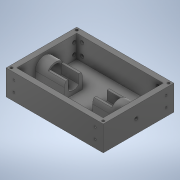
# Autodesk Inventor part: BodyWedgeBaseV3.1
Saved by Autodesk Inventor 2020 (Build 240168000, 168)
## iProperties
Created: 2023-11-26
Part Number: BodyWedgeBaseV3.1
Material: Thermoplastic Resin
Document SubType Name: Modeling
Designer: smz3rm
Density: 1.28 g/cm^3
Appearance: Smooth - Black
Mass: 119.612 g
Surface Area: 420.017 cm^2
Volume: 93.4466 cm^3
SideThickness: 6.000 mm
BaseThickness: 3.000 mm
TopThickness: 1.588 mm
BoxWidth: 110.000 mm
BoxLength: 80.000 mm
Height: 30.000 mm
DriveMotorHeight: 15.000 mm
DriveMotorMountThickness: 2.000 mm
ScrewDia: 2.900 mm
ScrewDepth: 7.000 mm
ForkScrewHeadDia: 4.000 mm
ForkScrewDia: 2.200 mm
ForkScrewHeadDepth: 2.200 mm
DriveMotorOffset: 37.250 mm
DriveMotorDia: 16.500 mm
SideArmorWidth: 15.000 mm
ForkLength: 60.000 mm
WheelWidth: 16.510 mm
DriveMotorHoleDia: 3.500 mm
ForkPlugDia: 3.500 mm
ForkPlugTolerance: 0.500 mm
ForkPlugLength: 3.000 mm
Author: smz3rm
Autodesk Inventor part; units mm, degrees
ref_plane "YZ Plane" through (0, 0, 0) normal (1, 0, 0) x (0, 1, 0)
ref_plane "XZ Plane" through (0, 0, 0) normal (0, 1, 0) x (-1, 0, 0)
ref_plane "XY Plane" through (0, 0, 0) normal (0, 0, 1) x (1, 0, 0)
sketch "Sketch1" plane through (0, 0, 0) normal (0, 1, 0) x (-1, 0, 0)
  line L0 (55, 40) -> (-55, 40)
  line L1 (-55, 40) -> (-55, -40)
  line L2 (-55, -40) -> (55, -40)
  line L3 (55, -40) -> (55, 40)
  line L4 (55, 40) -> (-55, -40) construction
  line L5 (-55, 40) -> (55, -40) construction
  line L6 (0, -56) -> (0, 56) projected
  point P0 (0, 0)
  dimension "d0" = 110
  dimension "d1" = 80
  constraints: 12 end point, 2 midpoint, 2 parallel, 1 horizontal, 1 perpendicular
  measures "d0" distance of L2.end L1.end
  measures "d1" distance of L1.end L0.end
extrude "Extrusion1" add sketch "Sketch1" along normal blind 3
sketch "Sketch2" plane through (0, 3, 0) normal (0, 1, 0) x (1, 0, 0)
  line L0 (-55, 40) -> (-55, -40) projected
  line L1 (-55, -40) -> (55, -40) projected
  line L2 (55, -40) -> (55, 40) projected
  line L3 (49, -34) -> (-49, -34)
  line L4 (-49, -34) -> (-49, 34)
  line L5 (-49, 34) -> (49, 34)
  line L6 (49, 34) -> (49, -34)
  line L7 (49, -34) -> (-49, 34) construction
  line L8 (-49, -34) -> (49, 34) construction
  line L9 (55, 40) -> (-55, 40) projected
  point P0 (0, 0)
  dimension "d36" = 98
  dimension "d37" = 68
  constraints: 12 end point, 2 midpoint, 2 parallel, 1 horizontal, 1 perpendicular
  measures "d36" distance of L4.end L5.end
  measures "d37" distance between parallel lines of L5 L3
extrude "Extrusion2" add sketch "Sketch2" along normal blind 25.4125
sketch "Sketch7" plane through (-49, 3, 34) normal (1, 0, 0) x (0, 0, -1)
  circle A0 centre (31.25, 12) radius 8.25
  line L0 (74, -3) -> (-6, -3) projected
  circle A1 centre (31.25, 12) radius 10.25
  line L1 (21, 12) -> (41.5, 12)
  line L2 (41.5, 12) -> (41.5, 0)
  line L3 (-6, -3) -> (-6, 25.4125) projected
  line L4 (0, 0) -> (41.5, 0)
  line L5 (0, 0) -> (0, 25.4125) projected
  line L6 (21, 12) -> (21, 0)
  line L7 (68, 0) -> (0, 0) projected
  point P0 (34, -3)
  point P1 (54, -3)
  point P2 (0, 25.25)
  point P3 (22.1693, 16.7543)
  point P4 (23, 12)
  point P5 (39.5, 12)
  dimension "MotorDiameter" = 16.5
  dimension "d18" = 15
  dimension "d20" = 2
  dimension "d144" = 37.25
  constraints: 8 end point, 3 point on circle, 2 centre point, 2 horizontal, 1 perpendicular, 1 point on line, 1 tangent, 1 vertical, 2 other
  measures "MotorDiameter" diameter of A0
  measures "d18" distance from line of L0 A0.centre
  measures "d20" radial gap between concentric circles of A0 A1
  measures "d144" horizontal distance of L0.end A0.centre
extrude "Extrusion5" add sketch "Sketch7" along normal blind 13 contours L1 A1 A0 | A0 L1 A1 | L2 L4 L6 A1
sketch "Sketch8" plane through (-36, 3, 34) normal (1, 0, 0) x (0, 0, -1)
  arc A0 (41.5, 12) -> (21, 12) centre (31.25, 12) ccw projected
  arc A1 (41.5, 12) -> (21, 12) centre (31.25, 12) ccw projected
  arc A2 (23, 12) -> (23, 12) centre (31.25, 12) ccw projected
  line L0 (41.5, 0) -> (21, 0) projected
  line L1 (21, 12) -> (21, 0) projected
  line L2 (41.5, 0) -> (21, 0) projected
  line L3 (41.5, 0) -> (41.5, 12) projected
  circle A3 centre (31.25, 12) radius 7.75
  line L4 (25.15, 17.5545) -> (25.15, 0)
  line L5 (31.25, 19.75) -> (31.25, 4.25)
  line L6 (37.35, 17.5545) -> (37.35, 0)
  circle A4 centre (31.25, 12) radius 8.25 projected
  arc A5 (41.5, 12) -> (21, 12) centre (31.25, 12) ccw projected
  line L7 (21, 12) -> (21, 0) projected
  line L8 (41.5, 0) -> (21, 0) projected
  line L9 (41.5, 0) -> (41.5, 12) projected
  line L10 (37.35, 17.5545) -> (39.8645, 17.5545)
  line L11 (25.15, 17.5545) -> (22.6355, 17.5545)
  point P0 (34, -3)
  point P1 (19.75, 15)
  point P2 (37.35, 7.2196)
  point P3 (25.15, 7.2196)
  point P4 (22.6355, 17.5545)
  dimension "d145" = 15.5
  dimension "d146" = 15.5
  dimension "d147" = 12.2
  constraints: 10 end point, 4 point on circle, 2 horizontal, 2 symmetric about line, 1 centre point, 1 coincident, 1 perpendicular, 1 point on line, 1 vertical, 2 other
  measures "d145" diameter of A3
  measures "d146" distance of L5.start L5.end
  measures "d147" distance between parallel lines of L4 L6
extrude "Extrusion6" add sketch "Sketch8" along normal blind 20 contours L3 L0 L6 A2 L10 A0 | L11 A2 L4 L0 L1 A0 | A2 L6 A3 | L0 L4 A2 L6 | L4 A3 A2 | A3 L6 | A2 L4 A3 L6 | L4 A3 picked at (32.1563, 4.1687)
sketch "Sketch9" plane through (-49, 17, 8.75) normal (1, 0, 0) x (0, 0, -1)
  line L0 (48.75, -17) -> (-31.25, -17) projected
  line L1 (-31.25, -17) -> (-31.25, 11.4125) projected
  arc A0 (-0.1, 3.5545) -> (12.1, 3.5545) centre (6, -2) ccw projected
  arc A1 (12.1, 3.5545) -> (-0.1, 3.5545) centre (6, -2) ccw projected
  circle A2 centre (6, -2) radius 8.25 projected
  circle A3 centre (6, -2) radius 1.75
  point P0 (8.75, -17)
  point P1 (44, -20)
  dimension "d148" = 3.5
  constraints: 1 centre point, 1 coincident, 1 other
  measures "d148" diameter of A3
extrude "Extrusion7" cut sketch "Sketch9" against normal up to surface (6 mm away) contours A3
mirror "Mirror2" about plane through (0, 0, 0) normal (1, 0, 0) of "Extrusion7", "Extrusion6", "Extrusion5"
sketch "Sketch28" plane through (-49, 3, -34) normal (0, 0, 1) x (1, 0, 0)
  line L0 (98, 0) -> (0, 0) projected
  line L1 (98, 0) -> (98, 25.4125) projected
  line L2 (0, 0) -> (0, 25.4125) projected
  line L3 (92, 19.4125) -> (92, 6)
  line L4 (92, 6) -> (6, 6)
  line L5 (6, 6) -> (6, 19.4125)
  line L6 (6, 19.4125) -> (92, 19.4125)
  circle A0 centre (6, 19.4125) radius 2
  circle A1 centre (6, 6) radius 2
  circle A2 centre (92, 19.4125) radius 2
  circle A3 centre (92, 6) radius 2
  line L7 (0, 25.4125) -> (98, 25.4125) projected
  point P0 (49, -3)
  dimension "d120" = 4
  dimension "d121" = 4
  dimension "d122" = 4
  dimension "d123" = 4
  dimension "d132" = 6
  dimension "d133" = 6
  dimension "d134" = 6
  constraints: 8 end point, 4 centre point, 4 coincident, 2 other
  measures "d120" diameter of A0
  measures "d121" diameter of A1
  measures "d122" diameter of A2
  measures "d123" diameter of A3
  measures "d132" distance between parallel lines of L7 L6
  measures "d133" distance between parallel lines of L0 L4
  measures "d134" distance between parallel lines of L2 L5
extrude "Extrusion24" cut sketch "Sketch28" against normal blind 2.2 contours L6 A2 L3 | L3 A2 L6 | A3 L4 L3 | L3 L4 A3 | A0 L5 L6 | L6 L5 A0 | A1 L5 L4 | L4 L5 A1
sketch "Sketch29" plane through (-43, 22.4125, -36.2) normal (0, 0, 1) x (1, 0, 0)
  circle A0 centre (0, 0) radius 2 projected
  circle A1 centre (0, -13.4125) radius 2 projected
  circle A2 centre (86, 0) radius 2 projected
  circle A3 centre (86, -13.4125) radius 2 projected
  circle A4 centre (0, 0) radius 1.1
  circle A5 centre (0, -13.4125) radius 1.1
  circle A6 centre (86, 0) radius 1.1
  circle A7 centre (86, -13.4125) radius 2 projected
  circle A8 centre (86, -13.4125) radius 1.1
  point P0 (43, -22.4125)
  dimension "d126" = 2.2
  dimension "d127" = 2.2
  dimension "d128" = 2.2
  dimension "d129" = 2.2
  constraints: 4 centre point, 4 coincident
  measures "d126" diameter of A4
  measures "d127" diameter of A5
  measures "d128" diameter of A6
  measures "d129" diameter of A8
extrude "Extrusion25" cut sketch "Sketch29" against normal up to surface (3.8 mm away) contours A4 | A5 | A6 | A8
sketch "Sketch30" plane through (0, 28.4125, 0) normal (0, 1, 0) x (1, 0, 0)
  line L0 (-55, 40) -> (-55, -40) projected
  line L1 (-55, 37) -> (54.8299, 37)
  line L2 (55, 40) -> (-55, 40) projected
  line L3 (-52, 40) -> (-52, -40)
  line L4 (-55, -40) -> (55, -40) projected
  circle A0 centre (-52, 37) radius 1.45
  line L5 (-55, -37) -> (55, -37)
  circle A1 centre (-52, -37) radius 1.45
  point P0 (0, 0)
  dimension "d135" = 3
  dimension "d136" = 3
  dimension "d137" = 2.9
  dimension "d138" = 3
  dimension "d139" = 2.9
  constraints: 8 point on line, 6 end point, 2 centre point, 2 horizontal, 1 vertical
  measures "d135" distance of L0.start L1.start
  measures "d136" distance of L0.end L3.end
  measures "d137" diameter of A0
  measures "d138" distance of L0.end L5.start
  measures "d139" diameter of A1
extrude "Extrusion26" cut sketch "Sketch30" against normal blind 7 contours A0 L3 L1 | L1 L3 A0 | A0 L1 L3 | A1 L3 L5 | L5 L3 A1 | L1 A0 L3 | L5 A1 L3 | L3 A1 L5
mirror "Mirror11" about plane through (0, 0, 0) normal (1, 0, 0) of "Extrusion26"
sketch "Sketch31" plane through (49, 3, 34) normal (-1, 0, 0) x (0, 0, 1)
  line L0 (-21, 12) -> (-21, 0) projected
  line L1 (0, 0) -> (-21, 0) projected
  line L2 (0, 0) -> (0, 25.4125) projected
  line L3 (-68, 25.4125) -> (0, 25.4125) projected
  line L4 (-68, 0) -> (-68, 25.4125) projected
  line L5 (-41.5, 0) -> (-68, 0) projected
  line L6 (-41.5, 0) -> (-41.5, 12) projected
  arc A0 (-21, 12) -> (-41.5, 12) centre (-31.25, 12) ccw projected
  line L7 (-68, 25.4125) -> (0, 25.4125) projected
  line L8 (-65, 25.4125) -> (-65, 0)
  line L9 (-41.5, 0) -> (-68, 0) projected
  line L10 (-68, 0) -> (-68, 25.4125) projected
  circle A1 centre (-65, 18) radius 2
  circle A2 centre (-65, 6) radius 2
  point P0 (-34, -3)
  dimension "d150" = 3
  dimension "d152" = 4
  dimension "d153" = 7.4125
  dimension "d154" = 4
  dimension "d155" = 6
  constraints: 4 point on line, 2 centre point, 2 end point, 1 vertical
  measures "d150" distance between parallel lines of L4 L8
  measures "d152" diameter of A1
  measures "d153" distance of L8.start A1.centre
  measures "d154" diameter of A2
  measures "d155" distance from line of L5 A2.centre
extrude "Extrusion27" cut sketch "Sketch31" against normal blind 2.2 contours A2 L8 | L8 A2 | A1 L8 | L8 A1
sketch "Sketch32" plane through (51.2, 21, -31) normal (-1, 0, 0) x (0, 0, 1)
  circle A0 centre (0, 0) radius 2 projected
  circle A1 centre (0, 0) radius 2 projected
  circle A2 centre (0, -12) radius 2 projected
  circle A3 centre (0, -12) radius 2 projected
  circle A4 centre (0, 0) radius 1.1
  circle A5 centre (0, -12) radius 1.1
  point P0 (31, -21)
  dimension "d158" = 2.2
  dimension "d159" = 2.2
  constraints: 2 centre point, 2 coincident
  measures "d158" diameter of A4
  measures "d159" diameter of A5
extrude "Extrusion28" cut sketch "Sketch32" against normal up to surface (3.8 mm away) contours A4 | A5
sketch "Sketch33" plane through (49, 3, 34) normal (0, 0, -1) x (-1, 0, 0)
  line L0 (98, 0) -> (0, 0) projected
  line L1 (98, 0) -> (98, 25.4125) projected
  line L2 (0, 25.4125) -> (98, 25.4125) projected
  line L3 (0, 0) -> (0, 25.4125) projected
  line L4 (0, 25.4125) -> (98, 25.4125) projected
  line L5 (3, 25.4125) -> (3, 0)
  line L6 (98, 0) -> (0, 0) projected
  circle A0 centre (3, 18) radius 2
  circle A1 centre (3, 6) radius 2
  point P0 (49, -3)
  dimension "d162" = 3
  dimension "d163" = 4
  dimension "d164" = 4
  dimension "d165" = 7.4125
  dimension "d166" = 6
  constraints: 4 point on line, 2 centre point, 2 end point, 1 perpendicular
  measures "d162" distance between parallel lines of L3 L5
  measures "d163" diameter of A0
  measures "d164" diameter of A1
  measures "d165" distance of A0.centre L5.start
  measures "d166" distance of L5.end A1.centre
extrude "Extrusion29" cut sketch "Sketch33" against normal blind 2.2 contours A1 L5 | L5 A1 | A0 L5 | L5 A0
sketch "Sketch34" plane through (46, 21, 36.2) normal (0, 0, -1) x (-1, 0, 0)
  circle A0 centre (0, 0) radius 2 projected
  circle A1 centre (0, -12) radius 2 projected
  circle A2 centre (0, 0) radius 1.1
  circle A3 centre (0, -12) radius 1.1
  point P0 (46, -21)
  dimension "d169" = 2.2
  dimension "d170" = 2.2
  constraints: 2 centre point, 2 coincident
  measures "d169" diameter of A2
  measures "d170" diameter of A3
extrude "Extrusion30" cut sketch "Sketch34" against normal up to surface (3.8 mm away) contours A2 | A3
mirror "Mirror13" about plane through (0, 0, 0) normal (1, 0, 0) of "Extrusion27", "Extrusion28", "Extrusion29", "Extrusion30"
equation "\"d0\" = BoxWidth"
equation "\"d1\" = BoxLength"
equation "\"d2\" = BaseThickness"
equation "\"d37\" = BoxLength - 2 * SideThickness"
equation "\"d18\" = DriveMotorHeight"
equation "\"d20\" = DriveMotorMountThickness"
equation "\"SideThickness\" = 6"
equation "\"BaseThickness\" = 3"
equation "\"TopThickness\" = 1.5875"
equation "\"BoxWidth\" = 110"
equation "\"BoxLength\" = 80"
equation "\"Height\" = 30"
equation "\"DriveMotorHeight\" = 0.5 * Height"
equation "\"DriveMotorMountThickness\" = 2"
equation "\"ScrewDia\" = 2.9"
equation "\"ScrewDepth\" = 7"
equation "\"ForkScrewHeadDia\" = 4"
equation "\"ForkScrewDia\" = 2.2"
equation "\"ForkScrewHeadDepth\" = 2.2"
equation "\"DriveMotorOffset\" = 37.25"
equation "\"DriveMotorDia\" = 16.5"
equation "\"SideArmorWidth\" = 15"
equation "\"ForkLength\" = 60"
equation "\"WheelWidth\" = 16.51"
equation "\"DriveMotorHoleDia\" = 3.5"
equation "\"ForkPlugDia\" = 3.5"
equation "\"ForkPlugTolerance\" = 0.5"
equation "\"ForkPlugLength\" = 3"
body "Solid1"
